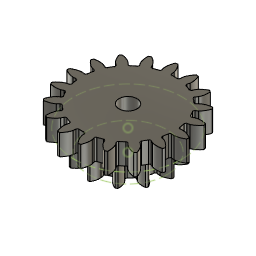
rear axle gear v5 (Autodesk Fusion 360 design; units mm, degrees)
description: Spur Gear; Module: 2.0; Num Teeth: 13; Pressure Angle: 20.0; Backlash: 1.00 mm
description: Spur Gear; Module: 2.0; Num Teeth: 18; Pressure Angle: 20.0; Backlash: 1.00 mm
Autodesk Fusion 360 part; units mm, degrees
sketch "Sketch1" plane through (0, 0, 0) normal (0, 0, 1) x (1, 0, 0) in component "Spur Gear (13 teeth)"
  circle A0 centre (0, 0) radius 10.5492
  circle A1 centre (0, 0) radius 3
extrude "Extrude1" add sketch "Sketch1" along normal blind 7 makes body 1 in component "Spur Gear (13 teeth)"
sketch "Sketch2" plane through (0, 0, 0) normal (0, 0, 1) x (1, 0, 0) in component "Spur Gear (13 teeth)"
  spline S0 degree 5 poles (12.1332, -1.42) (12.1414, -1.4209) (12.1578, -1.4226) (12.1824, -1.4243) (12.2153, -1.4252) (12.2566, -1.4243) (12.2979, -1.422) (12.3393, -1.4188) (12.3808, -1.4151) (12.4222, -1.4111) (12.4637, -1.4067) (12.5053, -1.4019) (12.5468, -1.3965) (12.5884, -1.3904) (12.6299, -1.3836) (12.6715, -1.3761) (12.7131, -1.3681) (12.7547, -1.3596) (12.7963, -1.3507) (12.8379, -1.3414) (12.8795, -1.3317) (12.9211, -1.3216) (12.9627, -1.311) (13.0042, -1.3001) (13.0458, -1.2886) (13.0873, -1.2768) (13.1288, -1.2645) (13.1703, -1.2519) (13.2118, -1.2389) (13.2533, -1.2255) (13.2947, -1.2118) (13.3361, -1.1977) (13.3775, -1.1833) (13.4188, -1.1684) (13.4602, -1.1533) (13.5015, -1.1378) (13.5427, -1.1219) (13.584, -1.1057) (13.6251, -1.0891) (13.6663, -1.0723) (13.7074, -1.0551) (13.7485, -1.0375) (13.7895, -1.0197) (13.8305, -1.0015) (13.8715, -0.983) (13.9124, -0.9642) (13.9533, -0.9451) (13.9941, -0.9257) (14.0349, -0.9059) (14.0756, -0.8859) (14.1162, -0.8656) (14.1569, -0.8449) (14.1974, -0.824) (14.2379, -0.8028) (14.2784, -0.7813) (14.3188, -0.7594) (14.3592, -0.7373) (14.3994, -0.7149) (14.4397, -0.6923) (14.4798, -0.6693) (14.5199, -0.6461) (14.56, -0.6226) (14.6, -0.5988) (14.6399, -0.5747) (14.6797, -0.5503) (14.7195, -0.5257) (14.7592, -0.5008) (14.7989, -0.4756) (14.8384, -0.4502) (14.8779, -0.4245) (14.9174, -0.3985) (14.9489, -0.3776) (14.9725, -0.3617) (14.9882, -0.3511) (14.996, -0.3458) knots 0 0 0 0 0 0 0.01428571 0.02857143 0.04285714 0.05714286 0.07142857 0.08571429 0.1 0.11428571 0.12857143 0.14285714 0.15714286 0.17142857 0.18571429 0.2 0.21428571 0.22857143 0.24285714 0.25714286 0.27142857 0.28571429 0.3 0.31428571 0.32857143 0.34285714 0.35714286 0.37142857 0.38571429 0.4 0.41428571 0.42857143 0.44285714 0.45714286 0.47142857 0.48571429 0.5 0.51428571 0.52857143 0.54285714 0.55714286 0.57142857 0.58571429 0.6 0.61428571 0.62857143 0.64285714 0.65714286 0.67142857 0.68571429 0.7 0.71428571 0.72857143 0.74285714 0.75714286 0.77142857 0.78571429 0.8 0.81428571 0.82857143 0.84285714 0.85714286 0.87142857 0.88571429 0.9 0.91428571 0.92857143 0.94285714 0.95714286 0.97142857 0.98571429 1 1 1 1 1 1
  spline S1 degree 5 poles (12.1332, 1.42) (12.1414, 1.4209) (12.1578, 1.4226) (12.1824, 1.4243) (12.2153, 1.4252) (12.2566, 1.4243) (12.2979, 1.422) (12.3393, 1.4188) (12.3808, 1.4151) (12.4222, 1.4111) (12.4637, 1.4067) (12.5053, 1.4019) (12.5468, 1.3965) (12.5884, 1.3904) (12.6299, 1.3836) (12.6715, 1.3761) (12.7131, 1.3681) (12.7547, 1.3596) (12.7963, 1.3507) (12.8379, 1.3414) (12.8795, 1.3317) (12.9211, 1.3216) (12.9627, 1.311) (13.0042, 1.3001) (13.0458, 1.2886) (13.0873, 1.2768) (13.1288, 1.2645) (13.1703, 1.2519) (13.2118, 1.2389) (13.2533, 1.2255) (13.2947, 1.2118) (13.3361, 1.1977) (13.3775, 1.1833) (13.4188, 1.1684) (13.4602, 1.1533) (13.5015, 1.1378) (13.5427, 1.1219) (13.584, 1.1057) (13.6251, 1.0891) (13.6663, 1.0723) (13.7074, 1.0551) (13.7485, 1.0375) (13.7895, 1.0197) (13.8305, 1.0015) (13.8715, 0.983) (13.9124, 0.9642) (13.9533, 0.9451) (13.9941, 0.9257) (14.0349, 0.9059) (14.0756, 0.8859) (14.1162, 0.8656) (14.1569, 0.8449) (14.1974, 0.824) (14.2379, 0.8028) (14.2784, 0.7813) (14.3188, 0.7594) (14.3592, 0.7373) (14.3994, 0.7149) (14.4397, 0.6923) (14.4798, 0.6693) (14.5199, 0.6461) (14.56, 0.6226) (14.6, 0.5988) (14.6399, 0.5747) (14.6797, 0.5503) (14.7195, 0.5257) (14.7592, 0.5008) (14.7989, 0.4756) (14.8384, 0.4502) (14.8779, 0.4245) (14.9174, 0.3985) (14.9489, 0.3776) (14.9725, 0.3617) (14.9882, 0.3511) (14.996, 0.3458) knots 0 0 0 0 0 0 0.01428571 0.02857143 0.04285714 0.05714286 0.07142857 0.08571429 0.1 0.11428571 0.12857143 0.14285714 0.15714286 0.17142857 0.18571429 0.2 0.21428571 0.22857143 0.24285714 0.25714286 0.27142857 0.28571429 0.3 0.31428571 0.32857143 0.34285714 0.35714286 0.37142857 0.38571429 0.4 0.41428571 0.42857143 0.44285714 0.45714286 0.47142857 0.48571429 0.5 0.51428571 0.52857143 0.54285714 0.55714286 0.57142857 0.58571429 0.6 0.61428571 0.62857143 0.64285714 0.65714286 0.67142857 0.68571429 0.7 0.71428571 0.72857143 0.74285714 0.75714286 0.77142857 0.78571429 0.8 0.81428571 0.82857143 0.84285714 0.85714286 0.87142857 0.88571429 0.9 0.91428571 0.92857143 0.94285714 0.95714286 0.97142857 0.98571429 1 1 1 1 1 1
  arc A0 (14.996, -0.3458) -> (14.996, 0.3458) centre (0, 0) ccw
  line L0 (10.4678, -1.2262) -> (12.1332, -1.42)
  line L1 (10.4678, 1.2262) -> (12.1332, 1.42)
  line L2 (10.4678, -1.2262) -> (10.4678, 1.2262)
  point P0 (12.3335, -1.4191)
  point P1 (12.536, -1.3978)
  point P2 (12.7399, -1.3625)
  point P3 (12.9448, -1.3155)
  point P4 (13.1503, -1.258)
  point P5 (13.3562, -1.1907)
  point P6 (13.5623, -1.1141)
  point P7 (13.7685, -1.0288)
  point P8 (13.9745, -0.935)
  point P9 (14.1801, -0.8329)
  point P10 (14.3853, -0.7228)
  point P11 (14.5898, -0.6048)
  point P12 (14.7934, -0.4791)
  point P13 (12.3335, 1.4191)
  point P14 (12.536, 1.3978)
  point P15 (12.7399, 1.3625)
  point P16 (12.9448, 1.3155)
  point P17 (13.1503, 1.258)
  point P18 (13.3562, 1.1907)
  point P19 (13.5623, 1.1141)
  point P20 (13.7685, 1.0288)
  point P21 (13.9745, 0.935)
  point P22 (14.1801, 0.8329)
  point P23 (14.3853, 0.7228)
  point P24 (14.5898, 0.6048)
  point P25 (14.7934, 0.4791)
extrude "Extrude2" add sketch "Sketch2" along normal blind 7 bodies 1 in component "Spur Gear (13 teeth)"
fillet "Fillet1" radius 0.5 2 edges at (10.4776, -1.2274, 3.5) (10.4776, 1.2274, 3.5) on bodies 1 in component "Spur Gear (13 teeth)"
pattern_circular "C-Pattern1" count 13 over 360 about axis through (0, 0, 0) along (0, 0, 1) of "Extrude2", "Fillet1" in component "Spur Gear (13 teeth)"
sketch "Sketch3" plane through (0, 0, 0) normal (0, 0, 1) x (1, 0, 0) in component "Spur Gear (13 teeth)"
  circle A0 centre (0, 0) radius 13 construction
sketch "Sketch1 (2)" plane through (0, 0, 0) normal (0, 0, 1) x (1, 0, 0) in component "Spur Gear (18 teeth)"
  circle A0 centre (0, 0) radius 15.5492
  circle A1 centre (0, 0) radius 3
extrude "Extrude1'" add sketch "Sketch1 (2)" along normal blind 7 separate body makes body 2 in component "Spur Gear (18 teeth)"
sketch "Sketch2 (2)" plane through (0, 0, 0) normal (0, 0, 1) x (1, 0, 0) in component "Spur Gear (18 teeth)"
  spline S0 degree 5 poles (16.8486, -1.4913) (16.8576, -1.4921) (16.8758, -1.4934) (16.9029, -1.4947) (16.9392, -1.495) (16.9846, -1.4934) (17.0301, -1.4904) (17.0756, -1.4866) (17.1212, -1.4823) (17.1668, -1.4776) (17.2123, -1.4726) (17.2579, -1.4672) (17.3035, -1.4612) (17.3491, -1.4545) (17.3947, -1.4471) (17.4403, -1.4391) (17.486, -1.4305) (17.5316, -1.4215) (17.5772, -1.4121) (17.6227, -1.4023) (17.6683, -1.3922) (17.7139, -1.3816) (17.7594, -1.3706) (17.805, -1.3592) (17.8505, -1.3474) (17.896, -1.3352) (17.9415, -1.3226) (17.987, -1.3096) (18.0324, -1.2962) (18.0778, -1.2825) (18.1232, -1.2685) (18.1686, -1.2541) (18.214, -1.2394) (18.2593, -1.2243) (18.3046, -1.2089) (18.3498, -1.1931) (18.3951, -1.177) (18.4403, -1.1606) (18.4855, -1.1439) (18.5306, -1.1268) (18.5757, -1.1095) (18.6208, -1.0918) (18.6658, -1.0739) (18.7108, -1.0556) (18.7558, -1.037) (18.8007, -1.0181) (18.8456, -0.999) (18.8904, -0.9795) (18.9352, -0.9598) (18.98, -0.9397) (19.0247, -0.9194) (19.0694, -0.8988) (19.114, -0.8779) (19.1586, -0.8567) (19.2031, -0.8353) (19.2476, -0.8135) (19.292, -0.7916) (19.3364, -0.7693) (19.3808, -0.7468) (19.4251, -0.724) (19.4693, -0.7009) (19.5135, -0.6776) (19.5576, -0.654) (19.6017, -0.6301) (19.6457, -0.606) (19.6897, -0.5816) (19.7336, -0.557) (19.7775, -0.5321) (19.8213, -0.507) (19.865, -0.4816) (19.9087, -0.4559) (19.9436, -0.4352) (19.9698, -0.4196) (19.9872, -0.4091) (19.9959, -0.4039) knots 0 0 0 0 0 0 0.01428571 0.02857143 0.04285714 0.05714286 0.07142857 0.08571429 0.1 0.11428571 0.12857143 0.14285714 0.15714286 0.17142857 0.18571429 0.2 0.21428571 0.22857143 0.24285714 0.25714286 0.27142857 0.28571429 0.3 0.31428571 0.32857143 0.34285714 0.35714286 0.37142857 0.38571429 0.4 0.41428571 0.42857143 0.44285714 0.45714286 0.47142857 0.48571429 0.5 0.51428571 0.52857143 0.54285714 0.55714286 0.57142857 0.58571429 0.6 0.61428571 0.62857143 0.64285714 0.65714286 0.67142857 0.68571429 0.7 0.71428571 0.72857143 0.74285714 0.75714286 0.77142857 0.78571429 0.8 0.81428571 0.82857143 0.84285714 0.85714286 0.87142857 0.88571429 0.9 0.91428571 0.92857143 0.94285714 0.95714286 0.97142857 0.98571429 1 1 1 1 1 1
  spline S1 degree 5 poles (16.8486, 1.4913) (16.8576, 1.4921) (16.8758, 1.4934) (16.9029, 1.4947) (16.9392, 1.495) (16.9846, 1.4934) (17.0301, 1.4904) (17.0756, 1.4866) (17.1212, 1.4823) (17.1668, 1.4776) (17.2123, 1.4726) (17.2579, 1.4672) (17.3035, 1.4612) (17.3491, 1.4545) (17.3947, 1.4471) (17.4403, 1.4391) (17.486, 1.4305) (17.5316, 1.4215) (17.5772, 1.4121) (17.6227, 1.4023) (17.6683, 1.3922) (17.7139, 1.3816) (17.7594, 1.3706) (17.805, 1.3592) (17.8505, 1.3474) (17.896, 1.3352) (17.9415, 1.3226) (17.987, 1.3096) (18.0324, 1.2962) (18.0778, 1.2825) (18.1232, 1.2685) (18.1686, 1.2541) (18.214, 1.2394) (18.2593, 1.2243) (18.3046, 1.2089) (18.3498, 1.1931) (18.3951, 1.177) (18.4403, 1.1606) (18.4855, 1.1439) (18.5306, 1.1268) (18.5757, 1.1095) (18.6208, 1.0918) (18.6658, 1.0739) (18.7108, 1.0556) (18.7558, 1.037) (18.8007, 1.0181) (18.8456, 0.999) (18.8904, 0.9795) (18.9352, 0.9598) (18.98, 0.9397) (19.0247, 0.9194) (19.0694, 0.8988) (19.114, 0.8779) (19.1586, 0.8567) (19.2031, 0.8353) (19.2476, 0.8135) (19.292, 0.7916) (19.3364, 0.7693) (19.3808, 0.7468) (19.4251, 0.724) (19.4693, 0.7009) (19.5135, 0.6776) (19.5576, 0.654) (19.6017, 0.6301) (19.6457, 0.606) (19.6897, 0.5816) (19.7336, 0.557) (19.7775, 0.5321) (19.8213, 0.507) (19.865, 0.4816) (19.9087, 0.4559) (19.9436, 0.4352) (19.9698, 0.4196) (19.9872, 0.4091) (19.9959, 0.4039) knots 0 0 0 0 0 0 0.01428571 0.02857143 0.04285714 0.05714286 0.07142857 0.08571429 0.1 0.11428571 0.12857143 0.14285714 0.15714286 0.17142857 0.18571429 0.2 0.21428571 0.22857143 0.24285714 0.25714286 0.27142857 0.28571429 0.3 0.31428571 0.32857143 0.34285714 0.35714286 0.37142857 0.38571429 0.4 0.41428571 0.42857143 0.44285714 0.45714286 0.47142857 0.48571429 0.5 0.51428571 0.52857143 0.54285714 0.55714286 0.57142857 0.58571429 0.6 0.61428571 0.62857143 0.64285714 0.65714286 0.67142857 0.68571429 0.7 0.71428571 0.72857143 0.74285714 0.75714286 0.77142857 0.78571429 0.8 0.81428571 0.82857143 0.84285714 0.85714286 0.87142857 0.88571429 0.9 0.91428571 0.92857143 0.94285714 0.95714286 0.97142857 0.98571429 1 1 1 1 1 1
  arc A0 (19.9959, -0.4039) -> (19.9959, 0.4039) centre (0, 0) ccw
  line L0 (15.4787, -1.3709) -> (16.8486, -1.4913)
  line L1 (15.4787, 1.3709) -> (16.8486, 1.4913)
  line L2 (15.4787, -1.3709) -> (15.4787, 1.3709)
  point P0 (17.0702, -1.4869)
  point P1 (17.2935, -1.4624)
  point P2 (17.5179, -1.4242)
  point P3 (17.7429, -1.3746)
  point P4 (17.9684, -1.3148)
  point P5 (18.1942, -1.2457)
  point P6 (18.4203, -1.1678)
  point P7 (18.6463, -1.0816)
  point P8 (18.8722, -0.9874)
  point P9 (19.0979, -0.8854)
  point P10 (19.3232, -0.7759)
  point P11 (19.5481, -0.659)
  point P12 (19.7724, -0.535)
  point P13 (17.0702, 1.4869)
  point P14 (17.2935, 1.4624)
  point P15 (17.5179, 1.4242)
  point P16 (17.7429, 1.3746)
  point P17 (17.9684, 1.3148)
  point P18 (18.1942, 1.2457)
  point P19 (18.4203, 1.1678)
  point P20 (18.6463, 1.0816)
  point P21 (18.8722, 0.9874)
  point P22 (19.0979, 0.8854)
  point P23 (19.3232, 0.7759)
  point P24 (19.5481, 0.659)
  point P25 (19.7724, 0.535)
extrude "Extrude2'" add sketch "Sketch2 (2)" along normal blind 7 bodies 2 in component "Spur Gear (18 teeth)"
fillet "Fillet1'" radius 0.5 2 edges at (15.4886, -1.3718, 3.5) (15.4886, 1.3718, 3.5) on bodies 2 in component "Spur Gear (18 teeth)"
pattern_circular "C-Pattern1'" count 18 over 360 about axis through (0, 0, 0) along (0, 0, 1) of "Extrude2'", "Fillet1'" in component "Spur Gear (18 teeth)"
sketch "Sketch3 (2)" plane through (0, 0, 0) normal (0, 0, 1) x (1, 0, 0) in component "Spur Gear (18 teeth)"
  circle A0 centre (0, 0) radius 18 construction
combine "Combine1" operation add target body 2 tool bodies 1 body 1 seen with x (1, 0, 0) y (0, 1, 0) z (0, 0, 1) at (0, 0, -7) in component "Spur Gear (18 teeth)"
component "Spur Gear (13 teeth)" placed x (1, 0, 0) y (0, 1, 0) z (0, 0, 1) at (0, 0, 0)
component "Spur Gear (18 teeth)" placed x (1, 0, 0) y (0, 1, 0) z (0, 0, 1) at (0, 0, 7)
